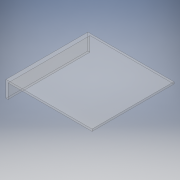
# Autodesk Inventor part: CameraMount
Saved by Autodesk Inventor 2017 (Build 210142000, 142)
## iProperties
Created: 2020-02-21
Part Number: CameraMount
Material: Polycarbonate, Clear
Document SubType Name: Modeling
Designer: S338674153
Density: 1.2 g/cm^3
Appearance: Polycarbonate - Clear
Author: S338674153
Autodesk Inventor part; units mm, degrees
ref_plane "YZ Plane" through (0, 0, 0) normal (1, 0, 0) x (0, 1, 0)
ref_plane "XZ Plane" through (0, 0, 0) normal (0, 1, 0) x (-1, 0, 0)
ref_plane "XY Plane" through (0, 0, 0) normal (0, 0, 1) x (1, 0, 0)
sketch "Sketch1" plane through (0, 0, 0) normal (0, 0, 1) x (1, 0, 0)
  line L0 (0, 0) -> (3.175, 0)
  line L1 (3.175, 0) -> (3.175, 22.225)
  line L2 (3.3662, 25.4) -> (0, 25.4)
  line L3 (0, 25.4) -> (0, 0)
  line L4 (0, 25.4) -> (133.35, 25.4)
  line L5 (133.35, 25.4) -> (133.35, 22.225)
  line L6 (133.35, 22.225) -> (3.175, 22.225)
  line L7 (0, 7.5436) -> (0, 25.4)
  dimension "d0" = 3.175
  dimension "d1" = 3.175
  dimension "d2" = 25.4
  dimension "d3" = 133.35
  constraints: 16 end point, 4 parallel, 2 horizontal, 2 perpendicular
  measures "d0" distance of L0.start L0.end
  measures "d1" distance of L4.end L5.end
  measures "d2" distance of L2.end L0.start
  measures "d3" distance of L2.end L4.end
extrude "Extrusion1" add sketch "Sketch1" along normal blind 127
body "Solid1"
